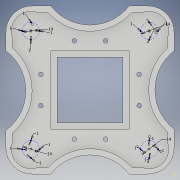
# Autodesk Inventor part: buttom_korpus
Saved by Autodesk Inventor 2019 (Build 230136000, 136)
## iProperties
Created: 2019-09-01
Part Number: buttom_korpus
Material: Типовые
Document SubType Name: Modeling
Designer: Professional
Density: 1 g/cm^3
Appearance: По умолчанию
Author: Professional
Autodesk Inventor part; units mm, degrees
ref_plane "YZ Plane" through (0, 0, 0) normal (1, 0, 0) x (0, 1, 0)
ref_plane "XZ Plane" through (0, 0, 0) normal (0, 1, 0) x (-1, 0, 0)
ref_plane "XY Plane" through (0, 0, 0) normal (0, 0, 1) x (1, 0, 0)
sketch "Эскиз1" plane through (0, 0, 0) normal (0, 0, 1) x (1, 0, 0)
  line L0 (0, 0) -> (-135, 0) construction
  line L1 (-135, 0) -> (-135, 135) construction
  line L2 (-135, 135) -> (0, 135) construction
  line L3 (0, 135) -> (0, 0) construction
  line L4 (-115, 115) -> (-20, 115) construction
  line L5 (-20, 115) -> (-20, 20) construction
  line L6 (-20, 20) -> (-115, 20) construction
  line L7 (-115, 20) -> (-115, 115) construction
  circle A0 centre (-115, 115) radius 10.75
  circle A1 centre (-20, 115) radius 10.75
  circle A2 centre (-115, 20) radius 10.75
  circle A3 centre (-20, 20) radius 10.75
  arc A4 (-114, 135) -> (-135, 114) centre (-114, 114) ccw
  arc A5 (0, 114) -> (-21, 135) centre (-21, 114) ccw
  arc A6 (-135, 20) -> (-114.0238, 0) centre (-114.0238, 21) ccw
  arc A7 (-21, 0) -> (0, 21) centre (-21, 21) ccw
  line L8 (-94, 94) -> (-41, 94) construction
  line L9 (-41, 94) -> (-41, 41) construction
  line L10 (-41, 41) -> (-94, 41) construction
  line L11 (-94, 41) -> (-94, 94) construction
  line L12 (-69, 94) -> (-66, 94) construction
  line L13 (-66, 94) -> (-66, 41) construction
  line L14 (-66, 41) -> (-69, 41) construction
  line L15 (-69, 41) -> (-69, 94) construction
  line L16 (-69, 49) -> (-66, 49) construction
  line L17 (-66, 49) -> (-66, 86) construction
  line L18 (-66, 86) -> (-69, 86) construction
  line L19 (-69, 86) -> (-69, 49) construction
  line L20 (-94, 94) -> (-94, 41)
  line L21 (-41, 41) -> (-94, 41)
  line L22 (-41, 94) -> (-41, 41)
  line L23 (-94, 94) -> (-41, 94)
  line L24 (-69, 49) -> (-66, 49)
  line L25 (-66, 86) -> (-69, 86)
  line L26 (-69, 49) -> (-94, 49)
  line L27 (-69, 86) -> (-94, 86)
  line L28 (-66, 86) -> (-41, 86)
  line L29 (-66, 49) -> (-41, 49)
  line L30 (-114.0238, 0) -> (-21, 0)
  line L31 (-135, 114) -> (-135, 20)
  line L32 (0, 21) -> (0, 114)
  line L33 (-21, 135) -> (-114, 135)
  dimension "d0" = 135
  dimension "d1" = 135
  dimension "d2" = 20
  dimension "d3" = 20
  dimension "d4" = 20
  dimension "d5" = 20
  dimension "d6" = 21.5
  dimension "d7" = 21.5
  dimension "d8" = 21.5
  dimension "d9" = 21.5
  dimension "d10" = 21
  dimension "d11" = 21
  dimension "d12" = 21
  dimension "d13" = 21
  dimension "d14" = 21
  dimension "d15" = 21
  dimension "d16" = 21
  dimension "d17" = 21
  dimension "d18" = 25
  dimension "d19" = 25
  dimension "d20" = 45
  dimension "d21" = 45
  constraints: 68 end point, 19 point on line, 10 parallel, 9 perpendicular, 8 centre point, 8 collinear, 8 point on circle, 8 tangent, 5 horizontal, 4 coincident
  measures "d0" distance of L1.end L2.end
  measures "d1" distance of L0.end L1.end
  measures "d2" distance between parallel lines of L2 L4
  measures "d3" distance from line of L0 L5.end
  measures "d4" distance from line of L1 L6.end
  measures "d5" distance from line of L3 L4.end
  measures "d6" diameter of A3
  measures "d7" diameter of A2
  measures "d8" diameter of A1
  measures "d9" diameter of A0
  measures "d10" radius of A6
  measures "d11" radius of A7
  measures "d12" radius of A4
  measures "d13" radius of A5
  measures "d14" distance between parallel lines of L4 L8
  measures "d15" distance between parallel lines of L11 L7
  measures "d16" distance between parallel lines of L6 L10
  measures "d17" distance between parallel lines of L5 L9
  measures "d18" distance between parallel lines of L15 L11
  measures "d19" distance between parallel lines of L13 L9
  measures "d20" distance between parallel lines of L16 L12
  measures "d21" distance between parallel lines of L10 L18
extrude "Выдавливание1" add sketch "Эскиз1" along normal blind 9
sketch "Эскиз2" plane through (0, 0, 9) normal (0, 0, 1) x (1, 0, 0)
  circle A0 centre (-115, 115) radius 10.75
  circle A1 centre (-115, 115) radius 10.75
  circle A2 centre (-20, 115) radius 10.75
  circle A3 centre (-20, 115) radius 10.75
  circle A4 centre (-115, 20) radius 10.75
  circle A5 centre (-115, 20) radius 10.75
  circle A6 centre (-20, 20) radius 10.75
  circle A7 centre (-20, 20) radius 10.75
  circle A8 centre (-20, 115) radius 1.5
  circle A9 centre (-115, 115) radius 1.5
  circle A10 centre (-115, 20) radius 1.5
  circle A11 centre (-20, 20) radius 1.5
  circle A12 centre (-115, 20) radius 10.75 projected
  circle A13 centre (-115, 115) radius 10.75 projected
  circle A14 centre (-20, 115) radius 10.75 projected
  circle A15 centre (-20, 20) radius 10.75 projected
  point P0 (0, 0)
  dimension "d24" = 3
  dimension "d25" = 3
  dimension "d26" = 3
  dimension "d27" = 3
  dimension "d111" = 21.5
  constraints: 12 centre point, 12 coincident, 4 concentric
  measures "d24" diameter of A8
  measures "d25" diameter of A9
  measures "d26" diameter of A10
  measures "d27" diameter of A11
  measures "d111" diameter of A4
extrude "Выдавливание2" add sketch "Эскиз2" against normal blind 9
sketch "Эскиз3" plane through (0, 0, 9) normal (0, 0, 1) x (1, 0, 0)
  circle A0 centre (-20, 20) radius 1.5 construction
  circle A1 centre (-20, 20) radius 7 construction
  circle A2 centre (-27, 20) radius 0.5
  circle A3 centre (-20, 27) radius 0.5
  circle A4 centre (-13, 20) radius 0.5
  circle A5 centre (-20, 13) radius 0.5
  circle A6 centre (-115, 20) radius 1.5 construction
  circle A7 centre (-115, 20) radius 7 construction
  circle A8 centre (-108, 20) radius 0.5
  circle A9 centre (-122, 20) radius 0.5
  circle A10 centre (-115, 27) radius 0.5
  circle A11 centre (-115, 13) radius 0.5
  circle A12 centre (-115, 115) radius 1.5 construction
  circle A13 centre (-115, 115) radius 7 construction
  circle A14 centre (-108, 115) radius 0.5
  circle A15 centre (-122, 115) radius 0.5
  circle A16 centre (-115, 122) radius 0.5
  circle A17 centre (-115, 108) radius 0.5
  circle A18 centre (-20, 115) radius 1.5 construction
  circle A19 centre (-20, 115) radius 7 construction
  circle A20 centre (-13, 115) radius 0.5
  circle A21 centre (-27, 115) radius 0.5
  circle A22 centre (-20, 122) radius 0.5
  circle A23 centre (-20, 108) radius 0.5
  point P0 (0, 0)
  dimension "d95" = 4
  dimension "d30" = 14
  dimension "d31" = 1
  dimension "d32" = 1
  dimension "d33" = 1
  dimension "d34" = 1
  dimension "d35" = 14
  dimension "d36" = 1
  dimension "d37" = 1
  dimension "d38" = 1
  dimension "d39" = 1
  dimension "d40" = 14
  dimension "d41" = 1
  dimension "d42" = 1
  dimension "d43" = 1
  dimension "d44" = 1
  dimension "d45" = 14
  dimension "d46" = 1
  dimension "d47" = 1
  dimension "d48" = 1
  dimension "d49" = 1
  constraints: 20 centre point, 16 point on circle, 8 horizontal alignment, 8 vertical alignment, 4 coincident
  measures "d30" diameter of A1
  measures "d31" diameter of A2
  measures "d32" diameter of A3
  measures "d33" diameter of A4
  measures "d34" diameter of A5
  measures "d35" diameter of A7
  measures "d36" diameter of A8
  measures "d37" diameter of A9
  measures "d38" diameter of A10
  measures "d39" diameter of A11
  measures "d40" diameter of A13
  measures "d41" diameter of A14
  measures "d42" diameter of A15
  measures "d43" diameter of A16
  measures "d44" diameter of A17
  measures "d45" diameter of A19
  measures "d46" diameter of A20
  measures "d47" diameter of A21
  measures "d48" diameter of A22
  measures "d49" diameter of A23
extrude "Выдавливание3" cut sketch "Эскиз3" against normal blind 9
sketch "Эскиз4" plane through (0, 0, 9) normal (0, 0, 1) x (1, 0, 0)
  line L0 (-135, 114) -> (-135, 20) projected
  arc A0 (-135, 35) -> (-135, 99) centre (-159, 67) ccw
  line L1 (-21, 135) -> (-114, 135) projected
  line L2 (0, 21) -> (0, 114) projected
  arc A1 (0, 99) -> (0, 36) centre (24.6526, 67.5) ccw
  line L3 (-114.0238, 0) -> (-21, 0) projected
  arc A2 (-99, 135) -> (-36, 135) centre (-67.5, 159.6526) ccw
  arc A3 (-36, 0) -> (-99.0238, 0) centre (-67.5119, -24.6374) ccw
  point P0 (0, 0)
  dimension "d52" = 15
  dimension "d53" = 15
  dimension "d56" = 15
  dimension "d57" = 15
  dimension "d61" = 15
  dimension "d62" = 15
  dimension "d63" = 40
  dimension "d64" = 40
  dimension "d65" = 40
  dimension "d108" = 15
  dimension "d109" = 15
  dimension "d110" = 40
  constraints: 8 point on circle, 8 point on line, 4 centre point
  measures "d52" distance of L2.end A1.start
  measures "d53" distance of L2.start A1.end
  measures "d56" distance of L0.end A0.start
  measures "d57" distance of L0.start A0.end
  measures "d61" distance of A2.start L1.end
  measures "d62" distance of L1.start A2.end
  measures "d63" radius of A2
  measures "d64" radius of A0
  measures "d65" radius of A1
  measures "d108" distance of A3.end L3.start
  measures "d109" distance of L3.end A3.start
  measures "d110" radius of A3
extrude "Выдавливание4" cut sketch "Эскиз4" against normal blind 12
shell "Оболочка1" thickness 5 removed faces 1 at (-32.3815, 68.8411, 9)
sketch "Эскиз5" plane through (0, 0, 9) normal (0, 0, 1) x (1, 0, 0)
  line L0 (-99, 99) -> (-99, 36) projected
  line L1 (-36, 36) -> (-99, 36)
  line L2 (-99, 36) -> (-99, 99)
  line L3 (-99, 99) -> (-36, 99)
  line L4 (-36, 99) -> (-36, 36)
  point P0 (0, 0)
  point P1 (-164, 109)
  constraints: 8 end point, 2 parallel, 1 horizontal, 1 perpendicular
sketch "Эскиз6" plane through (0, 0, 9) normal (0, 0, 1) x (1, 0, 0)
  circle A0 centre (-20, 20) radius 1.5 projected
  circle A1 centre (-20, 20) radius 15.75
  circle A2 centre (-20, 115) radius 1.5 projected
  circle A3 centre (-20, 115) radius 15.75
  circle A4 centre (-115, 20) radius 1.5 projected
  circle A5 centre (-115, 20) radius 15.75
  circle A6 centre (-115, 115) radius 1.5 projected
  circle A7 centre (-115, 115) radius 15.75
  point P0 (0, 0)
  dimension "d104" = 31.5
  dimension "d105" = 31.5
  constraints: 4 centre point, 4 coincident, 2 equal radius
  measures "d104" diameter of A3
  measures "d105" diameter of A7
extrude "Выдавливание6" cut sketch "Эскиз6" against normal blind 4
sketch "Эскиз7" plane through (0, 0, 0) normal (0, 0, -1) x (-1, 0, 0)
  circle A0 centre (28, 80) radius 2
  circle A1 centre (55, 107) radius 2
  circle A2 centre (80, 107) radius 2
  circle A3 centre (107, 80) radius 2
  circle A4 centre (107, 55) radius 2
  circle A5 centre (28, 55) radius 2
  circle A6 centre (20, 115) radius 10.75 projected
  line L0 (41, 41) -> (41, 94) projected
  line L1 (41, 94) -> (94, 94) projected
  line L2 (94, 94) -> (94, 41) projected
  arc A7 (36, 135) -> (99, 135) centre (67.5, 159.6526) ccw projected
  line L3 (41, 41) -> (41, 94) projected
  line L4 (94, 94) -> (94, 41) projected
  circle A8 centre (55, 28) radius 2
  circle A9 centre (80, 28) radius 2
  line L5 (94, 41) -> (41, 41) projected
  circle A10 centre (108, 20) radius 0.5 projected
  circle A11 centre (27, 20) radius 0.5 projected
  circle A12 centre (115, 108) radius 0.5 projected
  circle A13 centre (115, 115) radius 1.5 projected
  circle A14 centre (115, 20) radius 1.5 construction
  line L6 (20, 115) -> (115, 115) construction
  line L7 (115, 115) -> (115, 20) construction
  line L8 (115, 20) -> (20, 20) construction
  line L9 (20, 20) -> (20, 115) construction
  line L10 (67.5, 115) -> (67.5, 20) construction
  line L11 (20, 67.5) -> (115, 67.5) construction
  circle A15 centre (67.5, 67.5) radius 2.5
  point P0 (0, 0)
  point P1 (41, 114)
  point P2 (159, 114)
  point P3 (41, 86)
  point P4 (159, 86)
  dimension "d74" = 35
  dimension "d75" = 35
  dimension "d76" = 13
  dimension "d77" = 13
  dimension "d78" = 13
  dimension "d79" = 13
  dimension "d80" = 27
  dimension "d81" = 4
  dimension "d82" = 4
  dimension "d83" = 4
  dimension "d84" = 4
  dimension "d86" = 13
  dimension "d87" = 13
  dimension "d88" = 13
  dimension "d89" = 13
  dimension "d90" = 27
  dimension "d91" = 27
  dimension "d92" = 35
  dimension "d93" = 35
  dimension "d94" = 35
  dimension "d95" = 4
  dimension "d96" = 4
  dimension "d99" = 5
  dimension "d100" = 4
  dimension "d101" = 4
  constraints: 12 end point, 9 centre point, 5 midpoint, 2 parallel, 1 horizontal, 1 perpendicular, 2 other
  measures "d74" horizontal distance of L6.start A1.centre
  measures "d75" vertical distance of L6.start A0.centre
  measures "d76" distance from line of L0 A0.centre
  measures "d77" distance from line of L1 A1.centre
  measures "d78" distance from line of L1 A2.centre
  measures "d80" horizontal distance of A2.centre A3.centre
  measures "d81" diameter of A1
  measures "d82" diameter of A0
  measures "d83" diameter of A2
  measures "d84" diameter of A3
  measures "d86" distance from line of L3 A5.centre
  measures "d88" distance from line of L5 A8.centre
  measures "d89" distance from line of L5 A9.centre
  measures "d90" horizontal distance of A4.centre A9.centre
  measures "d91" horizontal distance of A5.centre A8.centre
  measures "d92" vertical distance of A10.centre A4.centre
  measures "d93" vertical distance of A11.centre A5.centre
  measures "d94" horizontal distance of A12.centre A2.centre
  measures "d95" diameter of A4
  measures "d96" diameter of A5
  measures "d99" diameter of A15
  measures "d100" diameter of A8
  measures "d101" diameter of A9
extrude "Выдавливание7" cut sketch "Эскиз7" against normal blind 10 contours A0 | A1 | A2 | A3 | A4 | A5 | A8 | A9 | A15
extrude "Выдавливание8" cut sketch "Эскиз5" against normal blind 6
